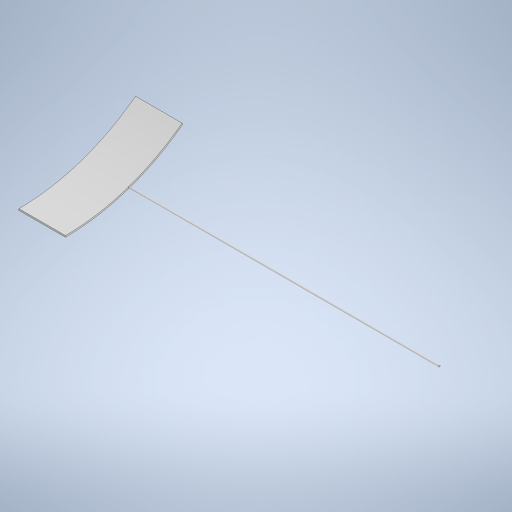
# Autodesk Inventor part: patch_antenna
Saved by Autodesk Inventor 2023 (Build 270158000, 158)
## iProperties
Created: 2023-05-21
Part Number: patch_antenna
Material: 一般
Document SubType Name: Modeling
Designer: 310611102
Density: 1 g/cm^3
Appearance: 預設
Author: 310611102
Autodesk Inventor part; units mm, degrees
ref_plane "YZ Plane" through (0, 0, 0) normal (1, 0, 0) x (0, 1, 0)
ref_plane "XZ Plane" through (0, 0, 0) normal (0, 1, 0) x (-1, 0, 0)
ref_plane "XY Plane" through (0, 0, 0) normal (0, 0, 1) x (1, 0, 0)
sketch "Sketch1" plane through (0, 0, 0) normal (1, 0, 0) x (0, 1, 0)
  arc A0 (-125, 0) -> (-99.8294, -75.2269) centre (0, 0) ccw
  line L0 (0, 0) -> (-126.6126, -95.4094)
  line L1 (0, 0) -> (-162.8559, 0)
  arc A1 (-126, 0) -> (-100.6281, -75.8287) centre (0, 0) ccw
  line L2 (-126, 0) -> (-125, 0)
  line L3 (-99.8294, -75.2269) -> (-100.6281, -75.8287)
  point P0 (-126, 0)
  point P1 (-100.6281, -75.8287)
  dimension "d0" = 250
  dimension "d1" = 37
  dimension "d2" = 1
  constraints: 8 end point, 5 point on circle, 2 centre point, 2 point on line, 1 coincident, 1 collinear, 1 horizontal
  measures "d0" diameter of A0
  measures "d1" angle of L1 L0
  measures "d2" radial gap between concentric circles of A0 A1
extrude "Extrusion1" add sketch "Sketch1" along normal blind 30 contours A0 L0 A1 L1
sketch "Sketch2" plane through (30, 0, 0) normal (1, 0, 0) x (0, 0, -1)
  circle A0 centre (41.1833, -118.5503) radius 0.5
  arc A1 (0, -125) -> (75.2269, -99.8294) centre (0, 0) ccw projected
  arc A2 (0, -126) -> (75.8287, -100.6281) centre (0, 0) ccw projected
  constraints: 2 tangent, 1 centre point
extrude "Extrusion2" add sketch "Sketch2" along normal blind 200
body "Solid1"
